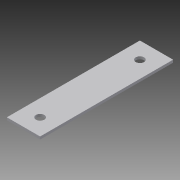
# Autodesk Inventor part: Part4
Saved by Autodesk Inventor 2013 (Build 170138000, 138)
## iProperties
Created: 2013-01-27
Part Number: Part4
Material: Aluminum 6061
Document SubType Name: Modeling
Designer: carneeki
Density: 1 g/cm^3
Author: carneeki
Autodesk Inventor part; units mm, degrees
ref_plane "YZ Plane" through (0, 0, 0) normal (1, 0, 0) x (0, 1, 0)
ref_plane "XZ Plane" through (0, 0, 0) normal (0, 1, 0) x (-1, 0, 0)
ref_plane "XY Plane" through (0, 0, 0) normal (0, 0, 1) x (1, 0, 0)
sketch "Sketch1" plane through (0, 0, 0) normal (0, 0, 1) x (1, 0, 0)
  line L0 (-12.7, 1) -> (12.7, 1)
  line L1 (12.7, 1) -> (12.7, -1)
  line L2 (12.7, -1) -> (-12.7, -1)
  line L3 (-12.7, -1) -> (-12.7, 1)
  point P0 (0, 0)
  dimension "d0" = 25.4
  dimension "d1" = 2
  dimension "d2" = 12.7
  dimension "d3" = 1
  constraints: 8 end point, 2 parallel, 1 horizontal, 1 perpendicular
  measures "d0" distance between parallel lines of L1 L3
  measures "d1" distance between parallel lines of L0 L2
  measures "d2" distance from line of point (0, 0) L1
  measures "d3" distance from line of point (0, 0) L0
extrude "Extrusion1" add sketch "Sketch1" against normal blind 101.6
sketch "Sketch2" plane through (-12.7, 1, 0) normal (0, 1, 0) x (1, 0, 0)
  line L0 (25.4, 0) -> (25.4, 101.6) projected
  line L1 (0, 101.6) -> (25.4, 101.6) projected
  circle A0 centre (12.7, 12.7) radius 2.5908
  circle A1 centre (12.7, 88.9) radius 2.5908
  point P0 (12.7, 0)
  dimension "d6" = 5.1816
  dimension "d7" = 12.7
  dimension "d8" = 12.7
  dimension "d9" = 5.1816
  dimension "d10" = 12.7
  constraints: 2 centre point, 1 vertical alignment
  measures "d6" diameter of A0
  measures "d7" distance from line of L0 A0.centre
  measures "d8" distance of point (12.7, 0) A0.centre
  measures "d9" diameter of A1
  measures "d10" distance from line of L1 A1.centre
hole "Hole1" at (0, 1, -88.9) at (0, 1, -12.7) direction (0, -1, 0) diameter 6.35 end through all
equation "\"d2\" = 0.5 * d0"
equation "\"d3\" = 0.5 * d1"
equation "\"d8\" = d7"
body "Solid1"
